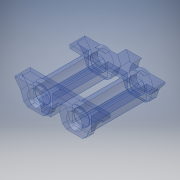
# Autodesk Inventor part: Holder
Saved by Autodesk Inventor 2019 (Build 230136000, 136)
## iProperties
Created: 2019-02-28
Part Number: Holder
Material: Woda
Document SubType Name: Modeling
Designer: atmat
Mass: 4.66349 g
Surface Area: 38.7698 cm^2
Volume: 4.67143 cm^3
Density: 0.9983 g/cm^3
Appearance: Tropikalnie niebieska
Author: atmat
Autodesk Inventor part; units mm, degrees
ref_plane "YZ Plane" through (0, 0, 0) normal (1, 0, 0) x (0, 1, 0)
ref_plane "XZ Plane" through (0, 0, 0) normal (0, 1, 0) x (-1, 0, 0)
ref_plane "XY Plane" through (0, 0, 0) normal (0, 0, 1) x (1, 0, 0)
sketch "Szkic1" plane through (0, 0, 0) normal (0, 1, 0) x (-1, 0, 0)
  line L0 (40.5, 28.01) -> (-40.5, 28.01)
  line L1 (-40.5, 28.01) -> (-40.5, 20)
  line L2 (-40.5, 20) -> (40.5, 20)
  line L3 (40.5, 20) -> (40.5, 28.01)
  line L4 (40.5, -20) -> (-40.5, -20)
  line L5 (-40.5, -20) -> (-40.5, -28.01)
  line L6 (-40.5, -28.01) -> (40.5, -28.01)
  line L7 (40.5, -28.01) -> (40.5, -20)
  point P0 (0, 0)
  dimension "d0" = 20
  dimension "d1" = 20
  dimension "d2" = 40.5
  dimension "d3" = 0
  dimension "d4" = 40.5
  dimension "d5" = 0
  dimension "d6" = 56.02
  dimension "d7" = 28.01
  constraints: 16 end point, 4 parallel, 2 horizontal, 2 perpendicular
  measures "d0" distance from line of point (0, 0) L2
  measures "d1" distance from line of point (0, 0) L4
  measures "d2" distance from line of point (0, 0) L3
  measures "d3" distance between parallel lines of L7 L3
  measures "d4" distance from line of point (0, 0) L1
  measures "d5" distance between parallel lines of L1 L5
  measures "d6" distance between parallel lines of L6 L0
  measures "d7" distance from line of point (0, 0) L0
extrude "Wyciągnięcie proste1" add sketch "Szkic1" along normal blind 3.6
sketch "Szkic2" plane through (40.5, 0, -28.01) normal (0, 0, -1) x (-1, 0, 0)
  line L0 (81, 3.6) -> (0, 3.6) projected
  line L1 (0, 3.6) -> (81, 3.6)
  line L2 (81, 3.6) -> (81, 2.025)
  line L3 (81, 2.025) -> (0, 2.025)
  line L4 (0, 2.025) -> (0, 3.6)
  line L5 (0, 0) -> (81, 0) projected
  point P0 (40.5, 0)
  dimension "d13" = 1.575
  constraints: 8 end point, 2 parallel, 1 horizontal, 1 perpendicular
  measures "d13" distance between parallel lines of L0 L3
extrude "Wyciągnięcie proste2" add sketch "Szkic2" along normal blind 7.29
mirror "Odbij1" about plane through (0, 0, 0) normal (0, 0, 1) of "Wyciągnięcie proste2"
sketch "Szkic3" plane through (40.5, 0, -35.3) normal (0, 0, -1) x (-1, 0, 0)
  circle A0 centre (20.85, -6) radius 8.025
  circle A1 centre (60.15, -6) radius 8.025
  line L0 (0, 2.025) -> (81, 2.025) projected
  point P0 (40.5, 0)
  dimension "d14" = 39.3
  dimension "d15" = 16.05
  dimension "d16" = 16.05
  dimension "d17" = 19.65
  dimension "d18" = 8.025
  dimension "d19" = 8.025
  constraints: 2 centre point
  measures "d14" distance of A1.centre A0.centre
  measures "d15" diameter of A0
  measures "d16" diameter of A1
  measures "d17" horizontal distance of point (40.5, 0) A0.centre
  measures "d18" distance from line of A0.centre L0
  measures "d19" distance from line of L0 A1.centre
extrude "Wyciągnięcie proste3" add sketch "Szkic3" against normal blind 7.29
mirror "Odbij2" about plane through (0, 0, 0) normal (0, 0, 1) of "Wyciągnięcie proste3"
sketch "Szkic4" plane through (40.5, 0, -35.3) normal (0, 0, -1) x (-1, 0, 0)
  circle A0 centre (20.85, -6) radius 11
  line L0 (81, 3.6) -> (0, 3.6) projected
  circle A1 centre (20.85, -6) radius 8.025 projected
  point P0 (40.5, 0)
  point P1 (20.85, 2.025)
  dimension "d22" = 22
  constraints: 1 centre point, 1 vertical alignment, 1 other
  measures "d22" diameter of A0
extrude "Wyciągnięcie proste4" add sketch "Szkic4" against normal blind 7.29
sketch "Szkic5" plane through (40.5, 0, -35.3) normal (0, 0, -1) x (-1, 0, 0)
  circle A0 centre (20.85, -6) radius 8.025
  arc A1 (15.5208, 0) -> (26.1792, 0) centre (20.85, -6) ccw projected
  point P0 (40.5, 0)
  dimension "d25" = 0
  constraints: 1 centre point, 1 concentric
  measures "d25" radial gap between concentric circles of A1 A0
extrude "Wyciągnięcie proste5" cut sketch "Szkic5" against normal blind 7.29
mirror "Odbij3" about plane through (0, 0, 0) normal (1, 0, 0) of "Wyciągnięcie proste5", "Wyciągnięcie proste4"
mirror "Odbij4" about plane through (0, 0, 0) normal (0, 0, 1) of "Wyciągnięcie proste5", "Wyciągnięcie proste4", "Odbij3"
sketch "Szkic6" plane through (40.5, 0, 20) normal (0, 0, -1) x (-1, 0, 0)
  line L0 (0, 3.6) -> (0, 2.025) projected
  line L1 (0, 3.6) -> (81, 3.6)
  line L2 (81, 3.6) -> (81, 5)
  line L3 (81, 5) -> (0, 5)
  line L4 (0, 5) -> (0, 3.6)
  line L5 (81, 2.025) -> (81, 3.6) projected
  arc A0 (65.5203, 3.6) -> (54.7797, 3.6) centre (60.15, -6) ccw projected
  point P0 (40.5, 0)
  dimension "d28" = 0
  dimension "d29" = 0
  constraints: 8 end point, 2 parallel, 1 horizontal, 1 perpendicular
  measures "d28" distance between parallel lines of L2 L5
  measures "d29" distance edge to line of A0 L3
extrude "Wyciągnięcie proste6" cut sketch "Szkic6" against normal blind 10 contours A0 L1
mirror "Odbij5" about plane through (0, 0, 0) normal (1, 0, 0) of "Wyciągnięcie proste6"
mirror "Odbij6" about plane through (0, 0, 0) normal (0, 0, 1) of "Wyciągnięcie proste6", "Odbij5"
sketch "Szkic7" plane through (40.5, 0, -35.3) normal (0, 0, -1) x (-1, 0, 0)
  arc A0 (11.6305, 0) -> (30.0695, 0) centre (20.85, -6) ccw projected
  line L0 (20.85, -17) -> (31.85, -17)
  arc A1 (52.6267, 2.025) -> (67.6733, 2.025) centre (60.15, -6) ccw projected
  line L1 (60.15, -17) -> (49.15, -17)
  line L2 (36, -5.4) -> (45, -5.4)
  line L3 (54.7797, 3.6) -> (26.2203, 3.6) projected
  line L4 (31.85, -17) -> (36, -5.4)
  line L5 (45, -5.4) -> (49.15, -17)
  line L6 (52.6267, 2.025) -> (28.3733, 2.025) projected
  arc A2 (20.85, -17) -> (28.3733, 2.025) centre (20.85, -6) ccw
  arc A3 (52.6267, 2.025) -> (60.15, -17) centre (60.15, -6) ccw
  line L7 (28.3733, 2.025) -> (52.6267, 2.025)
  line L8 (20.85, -17) -> (9.85, -17)
  line L9 (9.85, -17) -> (5.7, -5.4)
  line L10 (0, 0) -> (0, 3.6) projected
  line L11 (15.4797, 3.6) -> (0, 3.6) projected
  line L12 (60.15, -17) -> (71.15, -17)
  line L13 (71.15, -17) -> (75.3, -5.4)
  line L14 (81, 3.6) -> (65.5203, 3.6) projected
  line L15 (81, 0) -> (81, 3.6) projected
  line L16 (81, 2.025) -> (75.3, -5.4)
  line L17 (13.3267, 2.025) -> (0, 2.025) projected
  line L18 (5.7, -5.4) -> (0, 2.025)
  line L19 (0, 2.025) -> (13.3267, 2.025)
  arc A4 (13.3267, 2.025) -> (20.85, -17) centre (20.85, -6) ccw
  line L20 (67.6733, 2.025) -> (81, 2.025) projected
  arc A5 (60.15, -17) -> (67.6733, 2.025) centre (60.15, -6) ccw
  line L21 (67.6733, 2.025) -> (81, 2.025)
  point P0 (40.5, 0)
  dimension "d32" = 11
  dimension "d33" = 11
  dimension "d34" = 9
  dimension "d35" = 9
  dimension "d36" = 4.5
  dimension "d42" = 11
  dimension "d43" = 15.15
  dimension "d44" = 9
  dimension "d46" = 11
  dimension "d47" = 9
  dimension "d48" = 15.15
  dimension "d49" = 9.3606
  constraints: 28 end point, 10 point on circle, 9 tangent, 5 horizontal, 4 centre point, 3 concentric, 2 collinear, 2 point on line
  measures "d32" horizontal distance of A0.centre L0.end
  measures "d33" distance of L1.start L1.end
  measures "d34" distance between parallel lines of L3 L2
  measures "d35" distance of L2.start L2.end
  measures "d36" horizontal distance of L2.start point (40.5, 0)
  measures "d42" distance of L0.start L8.end
  measures "d43" horizontal distance of L9.end A0.centre
  measures "d44" distance from line of L11 L9.end
  measures "d46" distance of L1.start L12.end
  measures "d47" distance from line of L14 L13.end
  measures "d48" horizontal distance of L13.end A3.centre
  measures "d49" distance of L16.start L13.end
extrude "Wyciągnięcie proste7" add sketch "Szkic7" against normal blind 7.29
mirror "Odbij7" about plane through (0, 0, 0) normal (0, 0, 1) of "Wyciągnięcie proste7"
chamfer "Faza1" distance 3 angle 45 8 edges at (8.65, -17, -31.655) (8.65, -17, 31.655) (-8.65, -17, -31.655) (-8.65, -17, 31.655) (30.65, -17, -31.655) (-30.65, -17, -31.655) (-30.65, -17, 31.655) (30.65, -17, 31.655)
sketch "Szkic8" plane through (40.5, 0, -28.01) normal (0, 0, 1) x (1, 0, 0)
  line L0 (-16.1038, -12) -> (-25.5958, -12)
  arc A0 (-16.1038, -12) -> (-16.1038, 0) centre (-20.8496, -6) ccw
  arc A1 (-25.5958, 0) -> (-25.5958, -12) centre (-20.85, -6) ccw
  line L1 (-11.1996, -10.259) -> (-11.1996, 0)
  line L2 (-11.1996, 0) -> (-16.1038, 0)
  line L3 (-25.5958, 0) -> (-30.6194, 0)
  line L4 (-30.6194, 0) -> (-30.4172, -10.3219)
  line L5 (-11.1996, -10.259) -> (-11.1996, -15)
  line L6 (-11.1996, -15) -> (-30.3256, -15)
  line L7 (-30.3256, -15) -> (-30.4172, -10.3219)
  line L8 (-1.5545, 0) -> (-15.5208, 0) projected
  arc A2 (-26.1792, 0) -> (-15.5208, 0) centre (-20.85, -6) ccw projected
  point P0 (-40.5, 0)
  dimension "d50" = 9.492
  dimension "d51" = 9.492
  dimension "d52" = 0
  dimension "d53" = 7.65
  dimension "d54" = 7.65
  dimension "d55" = 9.65
  dimension "d56" = 2
  dimension "d57" = 3
  dimension "d58" = 12
  dimension "d59" = 0
  dimension "d60" = 0
  constraints: 16 end point, 4 point on circle, 2 centre point, 2 horizontal, 2 perpendicular, 2 vertical, 1 collinear
  measures "d50" distance of L0.start L0.end
  measures "d51" distance of L2.end L3.start
  measures "d52" horizontal distance of L2.end L0.start
  measures "d53" radius of A0
  measures "d54" radius of A1
  measures "d55" distance from line of L1 A0.centre
  measures "d56" distance edge to line of A1 L4
  measures "d57" distance between parallel lines of L6 L0
  measures "d58" distance between parallel lines of L2 L0
  measures "d59" distance between parallel lines of L8 L2
  measures "d60" distance of A2.centre A1.centre
extrude "Wyciągnięcie proste8" add sketch "Szkic8" along normal blind 28.01
chamfer "Faza2" distance 1 angle 45 4 edges at (10.1744, -15, -14.005) (9.8806, 0, -10) (29.3004, 0, -10) (29.3004, -15, -14.005)
mirror "Odbij8" about plane through (0, 0, 0) normal (1, 0, 0) of "Wyciągnięcie proste8", "Faza2"
mirror "Odbij9" about plane through (0, 0, 0) normal (0, 0, 1) of "Wyciągnięcie proste8", "Faza2", "Odbij8"
sketch "Szkic10" plane through (40.5, 0, -35.3) normal (0, 0, -1) x (-1, 0, 0)
  line L0 (32.8606, -14.1753) -> (36, -5.4) projected
  line L1 (36, -5.4) -> (45, -5.4) projected
  line L2 (36, -5.4) -> (45, -5.4)
  line L3 (54.7797, 3.6) -> (26.2203, 3.6) projected
  line L4 (48.1394, -14.1753) -> (45, -5.4) projected
  arc A0 (48.4145, 3.6) -> (45, -5.4) centre (60.15, -6) ccw
  arc A1 (36, -5.4) -> (32.5855, 3.6) centre (20.85, -6) ccw
  circle A2 centre (20.85, -6) radius 8.025 projected
  circle A3 centre (60.15, -6) radius 8.025 projected
  line L5 (32.5855, 3.6) -> (48.4145, 3.6)
  point P0 (40.5, 0)
  dimension "d67" = 0
  constraints: 4 end point, 4 point on circle, 2 centre point, 2 concentric, 1 collinear, 1 point on line
  measures "d67" distance from line of L5.start L3
extrude "Wyciągnięcie proste9" add sketch "Szkic10" along normal blind 9 contours A1 L3 A0 L1
mirror "Odbij10" about plane through (0, 0, 0) normal (0, 0, 1) of "Wyciągnięcie proste9"
